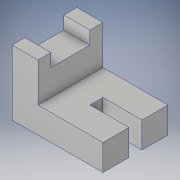
# Autodesk Inventor part: Aluminum Part
Saved by Autodesk Inventor 2017 (Build 210142000, 142)
## iProperties
Created: 2020-03-10
Part Number: Aluminum Part
Material: Aluminum 6061
Document SubType Name: Modeling
Designer: 10042265
Density: 2.7 g/cm^3
Appearance: Aluminum - Flat
Author: 10042265
Autodesk Inventor part; units mm, degrees
ref_plane "YZ Plane" through (0, 0, 0) normal (1, 0, 0) x (0, 1, 0)
ref_plane "XZ Plane" through (0, 0, 0) normal (0, 1, 0) x (-1, 0, 0)
ref_plane "XY Plane" through (0, 0, 0) normal (0, 0, 1) x (1, 0, 0)
sketch "Sketch1" plane through (0, 0, 0) normal (0, 0, 1) x (1, 0, 0)
  line L0 (0, 0) -> (44.45, 0)
  line L1 (44.45, 0) -> (44.45, 12.7)
  line L2 (44.45, 12.7) -> (12.7, 12.7)
  line L3 (12.7, 12.7) -> (12.7, 31.75)
  line L4 (12.7, 31.75) -> (0, 31.75)
  line L5 (0, 31.75) -> (0, 0)
  dimension "d0" = 44.45
  dimension "d1" = 12.7
  dimension "d2" = 31.75
  dimension "d3" = 19.05
  constraints: 12 end point, 5 perpendicular, 1 horizontal
  measures "d0" distance of L0.start L0.end
  measures "d1" distance of L0.end L1.end
  measures "d2" distance of L1.end L2.end
  measures "d3" distance of L2.end L3.end
extrude "Extrusion1" add sketch "Sketch1" along normal blind 31.75
sketch "Sketch2" plane through (0, 31.75, 0) normal (0, 1, 0) x (1, 0, 0)
  line L0 (0, -31.8326) -> (0, -25.4826) construction
  line L1 (0, 0) -> (0, -31.75) construction
  line L2 (0, -25.4826) -> (12.7, -25.4826)
  line L3 (12.7, 0) -> (12.7, -31.75) projected
  line L4 (12.7, -25.4826) -> (12.7, -6.4326)
  line L5 (12.7, -6.4326) -> (0, -6.4326)
  line L6 (0, -6.4326) -> (0, -25.4826)
  dimension "d6" = 6.35
  dimension "d7" = 19.05
  constraints: 10 end point, 4 point on line, 3 perpendicular
  measures "d6" distance of L0.start L0.end
  measures "d7" distance of L2.end L4.end
extrude "Extrusion2" cut sketch "Sketch2" against normal blind 6.35
sketch "Sketch4" plane through (12.7, 12.7, 0) normal (0, 1, 0) x (1, 0, 0)
  line L0 (31.75, 0) -> (31.75, -31.75) construction
  line L1 (31.75, -31.75) -> (31.75, -19.05) construction
  line L2 (31.75, -19.05) -> (12.7, -19.05)
  line L3 (12.7, -19.05) -> (12.7, -12.7)
  line L4 (12.7, -12.7) -> (31.75, -12.7)
  line L5 (31.75, -12.7) -> (31.75, -19.05)
  point P0 (-12.7, 0)
  dimension "d10" = 12.7
  dimension "d11" = 19.05
  dimension "d12" = 6.35
  constraints: 10 end point, 3 perpendicular, 2 point on line, 1 vertical
  measures "d10" distance of L0.end L1.end
  measures "d11" distance of L1.end L2.end
  measures "d12" distance of L2.end L3.end
extrude "Extrusion3" cut sketch "Sketch4" against normal blind 19.05
body "Solid1"
